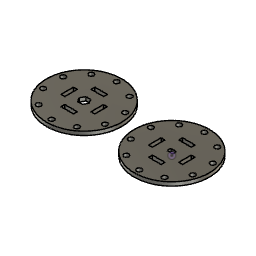
NEW Wheels (Autodesk Fusion 360 design; units mm, degrees)
Autodesk Fusion 360 part; units mm, degrees
sketch "Sketch1" plane through (0, 0, 0) normal (0, 0, 1) x (1, 0, 0)
  line L0 (0, 10.5) -> (5, 10.5)
  line L1 (5, 10.5) -> (5, 13.5)
  line L2 (5, 13.5) -> (-5, 13.5)
  line L3 (-5, 13.5) -> (-5, 10.5)
  line L4 (-5, 10.5) -> (0, 10.5)
  line L5 (10.5, 0) -> (10.5, 5)
  line L6 (10.5, 5) -> (13.5, 5)
  line L7 (13.5, 5) -> (13.5, -5)
  line L8 (13.5, -5) -> (10.5, -5)
  line L9 (10.5, -5) -> (10.5, 0)
  line L10 (0, -10.5) -> (5, -10.5)
  line L11 (5, -10.5) -> (5, -13.5)
  line L12 (5, -13.5) -> (-5, -13.5)
  line L13 (-5, -13.5) -> (-5, -10.5)
  line L14 (-5, -10.5) -> (0, -10.5)
  line L15 (-10.5, 0) -> (-10.5, 5)
  line L16 (-10.5, 5) -> (-13.5, 5)
  line L17 (-13.5, 5) -> (-13.5, -5)
  line L18 (-13.5, -5) -> (-10.5, -5)
  line L19 (-10.5, -5) -> (-10.5, 0)
  line L20 (0, 0) -> (0, 1.45)
  line L21 (0, 0) -> (0, -1.45)
  line L22 (0, -1.45) -> (-1.9748, -1.45)
  line L23 (1.9748, -1.45) -> (0, -1.45)
  line L24 (1.9748, 1.45) -> (-1.9748, 1.45)
  arc A0 (-1.9748, 1.45) -> (-1.9748, -1.45) centre (0, 0) ccw
  arc A1 (1.9748, -1.45) -> (1.9748, 1.45) centre (0, 0) ccw
  circle A2 centre (0, 0) radius 30
  circle A3 centre (0, 26) radius 2
  circle A4 centre (-15.2824, 21.0344) radius 2
  circle A5 centre (-24.7275, 8.0344) radius 2
  circle A6 centre (-24.7275, -8.0344) radius 2
  circle A7 centre (-15.2824, -21.0344) radius 2
  circle A8 centre (0, -26) radius 2
  circle A9 centre (15.2824, -21.0344) radius 2
  circle A10 centre (24.7275, -8.0344) radius 2
  circle A11 centre (24.7275, 8.0344) radius 2
  circle A12 centre (15.2824, 21.0344) radius 2
  line L25 (-80.5, -5) -> (-80.5, 0)
  circle A13 centre (-70, -26) radius 2
  line L26 (-80.5, 5) -> (-83.5, 5)
  line L27 (-75, -13.5) -> (-65, -13.5)
  circle A14 centre (-54.7176, -21.0344) radius 2
  line L28 (-75, -10.5) -> (-75, -13.5)
  circle A15 centre (-70, 26) radius 2
  circle A16 centre (-70, 0) radius 30
  circle A17 centre (-85.2824, 21.0344) radius 2
  line L29 (-83.5, -5) -> (-80.5, -5)
  circle A18 centre (-85.2824, -21.0344) radius 2
  line L30 (-56.5, -5) -> (-59.5, -5)
  line L31 (-56.5, 5) -> (-56.5, -5)
  line L32 (-75, 10.5) -> (-75, 13.5)
  line L33 (-70, -10.5) -> (-75, -10.5)
  line L34 (-70, 10.5) -> (-75, 10.5)
  circle A19 centre (-94.7275, -8.0344) radius 2
  line L35 (-80.5, 0) -> (-80.5, 5)
  circle A20 centre (-94.7275, 8.0344) radius 2
  line L36 (-83.5, 5) -> (-83.5, -5)
  line L37 (-75, 13.5) -> (-65, 13.5)
  line L38 (-65, 13.5) -> (-65, 10.5)
  circle A21 centre (-45.2725, 8.0344) radius 2
  line L39 (-65, -10.5) -> (-70, -10.5)
  circle A22 centre (-54.7176, 21.0344) radius 2
  line L40 (-59.5, 5) -> (-56.5, 5)
  line L41 (-65, 10.5) -> (-70, 10.5)
  line L42 (-65, -13.5) -> (-65, -10.5)
  circle A23 centre (-45.2725, -8.0344) radius 2
  line L43 (-59.5, -5) -> (-59.5, 0)
  line L44 (-59.5, 0) -> (-59.5, 5)
  line L45 (-71.9371, 3.3483) -> (-73.8682, -0.0035)
  line L46 (-73.8682, -0.0035) -> (-71.9311, -3.3517)
  line L47 (-71.9311, -3.3517) -> (-68.0629, -3.3483)
  line L48 (-68.0629, -3.3483) -> (-66.1318, 0.0035)
  line L49 (-66.1318, 0.0035) -> (-68.0689, 3.3517)
  line L50 (-68.0689, 3.3517) -> (-71.9371, 3.3483)
  point P0 (-70, 0)
  dimension "d4" = 10.5
  dimension "d5" = 5
  dimension "d6" = 3
  dimension "d7" = 10
  dimension "d8" = 3
  dimension "d9" = 10.5
  dimension "d10" = 5
  dimension "d11" = 3
  dimension "d12" = 10
  dimension "d13" = 3
  dimension "d14" = 10.5
  dimension "d15" = 5
  dimension "d16" = 3
  dimension "d17" = 10
  dimension "d18" = 3
  dimension "d19" = 10.5
  dimension "d20" = 5
  dimension "d21" = 3
  dimension "d22" = 10
  dimension "d23" = 3
  dimension "d37" = 4.9
  dimension "d38" = 1.45
  dimension "d39" = 1.45
  dimension "d42" = 60
  dimension "d44" = 4
  dimension "d46" = 360
  dimension "d47" = 3.35
  constraint perpendicular L0 L1
  constraint perpendicular L1 L2
  constraint perpendicular L0 L3
  constraint perpendicular L4 L5
  constraint perpendicular L4 L7
  constraint coincident L20.start L21.start
  constraint vertical L20
  constraint parallel L20 L21
  constraint perpendicular L21 L22
  constraint coincident L23.start A0
  constraint perpendicular L21 L23
  constraint perpendicular L20 L24
  constraint concentric A0 A1
  constraint coincident P0 A16.centre
  measures "d4" distance of L20.start L0.start
  measures "d5" distance of L0.start L0.end
  measures "d6" distance of L0.end L1.end
  measures "d7" distance of L1.end L2.end
  measures "d8" distance of L2.end L3.end
  measures "d9" distance of L20.start L5.start
  measures "d10" distance of L5.start L5.end
  measures "d11" distance of L5.end L6.end
  measures "d12" distance of L6.end L7.end
  measures "d13" distance of L7.end L8.end
  measures "d14" distance of L20.start L10.start
  measures "d15" distance of L10.start L10.end
  measures "d16" distance of L10.end L11.end
  measures "d17" distance of L11.end L12.end
  measures "d18" distance of L12.end L13.end
  measures "d19" distance of L20.start L15.start
  measures "d20" distance of L15.start L15.end
  measures "d21" distance of L15.end L16.end
  measures "d22" distance of L16.end L17.end
  measures "d23" distance of L17.end L18.end
  measures "d37" diameter of A0
  measures "d38" distance of L20.start L20.end
  measures "d39" distance of L20.start L21.end
  measures "d42" diameter of A2
  measures "d44" diameter of A3
  measures "d47" distance of P0 L50
sketch "Sketch2" plane through (0, 0, 0) normal (0, 0, 1) x (1, 0, 0)
sketch "Sketch3" plane through (0, 0, 0) normal (0, 0, 1) x (1, 0, 0)
extrude "Extrude1" add sketch "Sketch1" along normal blind 3 makes body 1 at (-81.0172, -12.5576, 0) makes body 2 at (-11.0172, -12.5576, 0)
